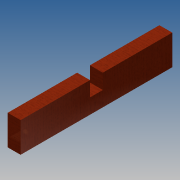
# Autodesk Inventor part: hubRingInnerWood
Saved by Autodesk Inventor 2014 SP1 (Build 180222100, 222)
## iProperties
Created: 2014-12-03
Part Number: hubRingInnerWood
Material: Wood (Oak)
Document SubType Name: Modeling
Designer: Dave
Mass: 1157.3 g
Surface Area: 1209.67 cm^2
Volume: 1522.77 cm^3
Density: 0.76 g/cm^3
Appearance: White Oak - Natural Medium Gloss
Author: Dave
Autodesk Inventor part; units mm, degrees
ref_plane "YZ Plane" through (0, 0, 0) normal (1, 0, 0) x (0, 1, 0)
ref_plane "XZ Plane" through (0, 0, 0) normal (0, 1, 0) x (-1, 0, 0)
ref_plane "XY Plane" through (0, 0, 0) normal (0, 0, 1) x (1, 0, 0)
sketch "Sketch1" plane through (0, 0, 0) normal (1, 0, 0) x (0, 1, 0)
  line L0 (0, 0) -> (88.9, 0)
  line L1 (88.9, 0) -> (88.9, -449.58)
  line L2 (88.9, -449.58) -> (0, -449.58)
  line L3 (0, -449.58) -> (0, 0)
  dimension "d0" = 88.9
  dimension "d1" = 449.58
  constraints: 8 end point, 2 parallel, 1 horizontal, 1 perpendicular
  measures "d0" distance of L1.end L2.end
  measures "d1" distance of L0.end L1.end
extrude "Extrusion1" add sketch "Sketch1" along normal blind 38.1
sketch "Sketch2" plane through (38.1, 0, 0) normal (1, 0, 0) x (0, 0, -1)
  line L0 (0, 88.9) -> (0, 0) projected
  line L1 (0, 0) -> (449.58, 0) projected
  line L2 (449.58, 88.9) -> (0, 88.9) projected
  line L3 (205.74, 88.9) -> (205.74, 44.45)
  line L4 (224.79, 88.9) -> (224.79, 0) construction
  line L5 (243.84, 88.9) -> (243.84, 44.45)
  line L6 (205.74, 44.45) -> (243.84, 44.45)
  line L7 (205.74, 88.9) -> (243.84, 88.9)
  dimension "d4" = 44.45
  dimension "d5" = 205.74
  constraints: 10 end point, 2 midpoint, 2 perpendicular, 2 symmetric about line, 1 collinear, 1 point on line
  measures "d4" distance of L3.start L3.end
  measures "d5" distance between parallel lines of L3 L0
extrude "Extrusion2" cut sketch "Sketch2" against normal blind 50.8
sketch "Sketch3" plane through (0, 0, -449.58) normal (0, -1, 0) x (1, 0, 0)
  line L0 (0, 0) -> (0, 449.58) projected
  line L1 (0, 0) -> (38.1, 0) projected
  line L2 (38.1, 449.58) -> (38.1, 0) projected
  line L3 (0, 449.58) -> (38.1, 449.58) projected
  line L4 (19.05, 449.58) -> (19.05, 0) construction
  line L5 (0, 224.79) -> (38.1, 224.79) construction
  circle A0 centre (19.05, 224.79) radius 7.9481
  constraints: 5 midpoint, 4 end point, 1 centre point
hole "Hole1" at (19.05, 0, -224.79) direction (0, 1, 0) diameter 6.35 depth 12.7 tip angle 118
body "Solid1"
